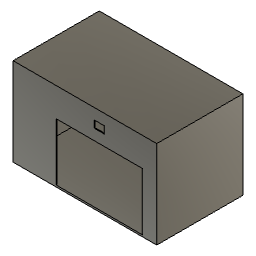
Parcelbox (Autodesk Fusion 360 design; units mm, degrees)
Autodesk Fusion 360 part; units mm, degrees
sketch "Onderkant" plane through (0, 0, 0) normal (0, 0, 1) x (1, 0, 0)
  line L0 (250, 150) -> (-250, 150)
  line L1 (-250, 150) -> (-250, -150)
  line L2 (-250, -150) -> (250, -150)
  line L3 (250, -150) -> (250, 150)
  line L4 (250, 150) -> (-250, -150) construction
  line L5 (-250, 150) -> (250, -150) construction
  dimension "d29" = 500
  dimension "d30" = 300
  constraint horizontal L0
  constraint perpendicular L0 L1
  constraint parallel L0 L2
  constraint parallel L1 L3
  constraint coincident L4 origin
  constraint coincident L5 origin
  measures "d29" distance of L1.end L2.end
  measures "d30" distance of L0.end L1.end
extrude "Extrude7" add sketch "Onderkant" along normal blind 6
sketch "Zijkanten" plane through (0, 0, 6) normal (0, 0, 1) x (-1, 0, 0)
  line L0 (-250, 150) -> (-250, -150)
  line L1 (-250, -150) -> (250, -150)
  line L2 (250, -150) -> (250, 150)
  line L3 (250, 150) -> (-250, 150)
  line L4 (-247, 147) -> (247, 147)
  line L5 (247, 147) -> (247, -147)
  line L6 (247, -147) -> (-247, -147)
  line L7 (-247, -147) -> (-247, 147)
  line L8 (-247, 147) -> (247, -147) construction
  line L9 (247, 147) -> (-247, -147) construction
  dimension "d33" = 494
  dimension "d34" = 294
  constraint horizontal L4
  constraint perpendicular L4 L5
  constraint parallel L4 L6
  constraint parallel L5 L7
  constraint coincident L8 origin
  constraint coincident L9 origin
  measures "d33" distance of L5.end L6.end
  measures "d34" distance of L4.end L5.end
extrude "Extrude8" add sketch "Zijkanten" along normal blind 300
sketch "Bovenkant" plane through (0, 0, 306) normal (0, 0, 1) x (-1, 0, 0)
  line L0 (247, -147) -> (-247, -147)
  line L1 (-247, -147) -> (-247, 147)
  line L2 (-247, 147) -> (247, 147)
  line L3 (247, 147) -> (247, -147)
  line L4 (250, 150) -> (-250, 150)
  line L5 (-250, 150) -> (-250, -150)
  line L6 (-250, -150) -> (250, -150)
  line L7 (250, -150) -> (250, 150)
  line L8 (-250, 150) -> (250, 150)
  line L9 (250, 150) -> (250, -150)
  line L10 (250, -150) -> (-250, -150)
  line L11 (-250, -150) -> (-250, 150)
  line L12 (-250, 150) -> (250, -150) construction
  line L13 (250, 150) -> (-250, -150) construction
  dimension "d37" = 500
  dimension "d38" = 300
  constraint horizontal L8
  constraint perpendicular L8 L9
  constraint parallel L8 L10
  constraint parallel L9 L11
  constraint coincident L12 origin
  constraint coincident L13 origin
  measures "d37" distance of L6.end L5.end
  measures "d38" distance of L4.start L6.end
extrude "Extrude9" add sketch "Bovenkant" against normal blind 6 contours L0 L1 L2 L3
sketch "Deur" plane through (0, -150, 0) normal (0, -1, 0) x (1, 0, 0)
  line L0 (-250, 0) -> (250, 0)
  line L1 (250, 0) -> (250, 306)
  line L2 (250, 306) -> (-250, 306)
  line L3 (-250, 306) -> (-250, 0)
  line L4 (200, 6) -> (-100, 6)
  line L5 (-100, 6) -> (-100, 206)
  line L6 (-100, 206) -> (200, 206)
  line L7 (200, 206) -> (200, 6)
  dimension "d42" = 300
  dimension "d43" = 200
  constraint horizontal L4
  constraint vertical L5
  constraint horizontal L6
  constraint vertical L7
  measures "d42" distance of L4.start L4.end
  measures "d43" distance of L4.start L6.end
extrude "Extrude10" cut sketch "Deur" against normal blind 6 contours L4 L5 L6 L7
sketch "Gat kabel" plane through (0, 150, 0) normal (0, 1, 0) x (-1, 0, 0)
  line L0 (-250, 0) -> (250, 0)
  line L1 (250, 0) -> (250, 306)
  line L2 (250, 306) -> (-250, 306)
  line L3 (-250, 306) -> (-250, 0)
  line L4 (240, 10) -> (220, 10)
  line L5 (220, 10) -> (220, 30)
  line L6 (220, 30) -> (240, 30)
  line L7 (240, 30) -> (240, 10)
  circle A0 centre (230, 20) radius 6
  dimension "d46" = 12
  constraint horizontal L4
  constraint vertical L5
  constraint horizontal L6
  constraint vertical L7
  measures "d46" diameter of A0
extrude "Extrude11" cut sketch "Gat kabel" against normal blind 6 contours A0
sketch "Gat scanner" plane through (0, -150, 0) normal (0, -1, 0) x (1, 0, 0)
  line L0 (-100, 6) -> (-100, 206)
  line L1 (-100, 206) -> (200, 206)
  line L2 (200, 206) -> (200, 6)
  line L3 (200, 6) -> (-100, 6)
  line L4 (-250, 0) -> (250, 0)
  line L5 (250, 0) -> (250, 306)
  line L6 (250, 306) -> (-250, 306)
  line L7 (-250, 306) -> (-250, 0)
  line L8 (67.5, 268.5) -> (32.5, 268.5)
  line L9 (32.5, 268.5) -> (32.5, 243.5)
  line L10 (32.5, 243.5) -> (67.5, 243.5)
  line L11 (67.5, 243.5) -> (67.5, 268.5)
  line L12 (67.5, 268.5) -> (32.5, 243.5) construction
  line L13 (32.5, 268.5) -> (67.5, 243.5) construction
  point P0 (50, 256)
  dimension "d51" = 35
  dimension "d52" = 25
  constraint horizontal L8
  constraint perpendicular L8 L9
  constraint parallel L8 L10
  constraint parallel L9 L11
  constraint coincident L12 P0
  constraint coincident L13 P0
  measures "d51" distance of L9.end L10.end
  measures "d52" distance of L8.end L9.end
extrude "Extrude12" cut sketch "Gat scanner" against normal blind 6 contours L8 L9 L10 L11
equation "lengte = 500 mm"
equation "breedte = 300 mm"
equation "hoogte = 300 mm"
equation "dikte_plaat = 6 mm"
equation "breedte_deur = 300 mm"
equation "hoogte_deur = 200 mm"
equation "d29 = lengte"
equation "d30 = breedte"
equation "d31 = dikte_plaat"
equation "d33 = lengte - dikte_plaat"
equation "d34 = breedte - dikte_plaat"
equation "d35 = hoogte"
equation "d37 = lengte"
equation "d38 = breedte"
equation "d39 = -dikte_plaat"
equation "d42 = breedte_deur"
equation "d43 = hoogte_deur"
equation "d44 = -dikte_plaat"
equation "d47 = -dikte_plaat"
equation "breedte_scanner = 35 mm"
equation "hoogte_scanner = 25 mm"
equation "d51 = breedte_scanner"
equation "d52 = hoogte_scanner"
equation "d53 = -dikte_plaat"
named bodies: "Parcelbox"
